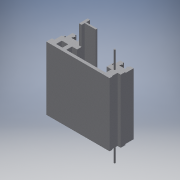
# Autodesk Inventor part: Platform
Saved by Autodesk Inventor 2016 (Build 200138000, 138)
## iProperties
Created: 2015-05-19
Part Number: Platform
Material: Steel
Document SubType Name: Modeling
Designer: Andy
Density: 7.85 g/cm^3
Appearance: Plate
Mass: 10057.4 g
Surface Area: 2204.12 cm^2
Volume: 1281.2 cm^3
Author: Andy
Autodesk Inventor part; units mm, degrees
ref_plane "YZ Plane" through (0, 0, 0) normal (1, 0, 0) x (0, 1, 0)
ref_plane "XZ Plane" through (0, 0, 0) normal (0, 1, 0) x (-1, 0, 0)
sketch "Sketch1" plane through (0, 0, 0) normal (0, 1, 0) x (-1, 0, 0)
  line L0 (0, 0) -> (199, 0)
  line L1 (199, 0) -> (199, 199)
  line L2 (199, 199) -> (0, 199)
  line L3 (0, 199) -> (0, 0)
  dimension "d0" = 199
  dimension "d1" = 199
  constraints: 8 end point, 2 parallel, 1 horizontal, 1 perpendicular
  measures "d0" distance of L0.start L0.end
  measures "d1" distance of L1.end L0.end
extrude "Extrusion1" add sketch "Sketch1" along normal blind 9
sketch "Sketch2" plane through (0, 9, 0) normal (0, 1, 0) x (1, 0, 0)
  line L0 (0, 0) -> (-199, 0) projected
  line L1 (-199, -199) -> (0, -199) projected
  line L2 (0, 0) -> (-2, 0)
  line L3 (-2, 0) -> (-2, -199)
  line L4 (-2, 0) -> (-21, 0)
  line L5 (-21, 0) -> (-21, -199)
  dimension "d4" = 2
  dimension "d5" = 19
  constraints: 8 end point, 4 point on line, 2 perpendicular
  measures "d4" distance of L0.start L2.end
  measures "d5" distance of L2.end L4.end
extrude "Extrusion2" add sketch "Sketch2" along normal blind 18
sketch "Sketch4" plane through (-199, 0, 199) normal (0, 0, 1) x (1, 0, 0)
  line L0 (178, 27) -> (197, 27) projected
  line L1 (197, 27) -> (207, 27)
  line L2 (207, 27) -> (207, 41)
  line L3 (178, 27) -> (163, 27)
  line L4 (163, 27) -> (163, 47)
  line L5 (163, 47) -> (165, 47)
  line L6 (165, 47) -> (165, 41)
  line L7 (165, 41) -> (207, 41)
  dimension "d9" = 10
  dimension "d10" = 14
  dimension "d11" = 15
  dimension "d12" = 20
  dimension "d13" = 2
  constraints: 14 end point, 5 perpendicular, 2 horizontal
  measures "d9" distance of L0.end L1.end
  measures "d10" distance of L1.end L2.end
  measures "d11" distance of L0.start L3.end
  measures "d12" distance of L3.end L4.end
  measures "d13" distance of L4.end L5.end
extrude "Extrusion3" add sketch "Sketch4" against normal blind 199
ref_plane "Work Plane1" through (-199, 0, 196) normal (0, 0, 1) x (1, 0, 0)
sketch "Sketch5" plane through (-199, 0, 196) normal (0, 0, 1) x (1, 0, 0)
  line L0 (165, 41) -> (207, 41)
  line L1 (207, 41) -> (207, 68)
  line L2 (165, 68) -> (165, 41)
  line L3 (176.05, 68) -> (176.05, 64.5)
  line L4 (176.05, 64.5) -> (180.3, 61.2)
  line L5 (195.95, 64.5) -> (191.7, 61.2)
  line L6 (195.95, 64.5) -> (195.95, 68)
  line L7 (195.95, 53) -> (195.95, 54.5)
  line L8 (195.95, 54.5) -> (191.7, 61.2)
  line L9 (176.05, 54.5) -> (180.3, 61.2)
  line L10 (176.05, 53) -> (176.05, 54.5)
  line L11 (195.95, 53) -> (176.05, 53)
  line L12 (207, 68) -> (195.95, 68)
  line L13 (207, 68) -> (195.95, 68)
  line L14 (176.05, 68) -> (165, 68)
  line L15 (15, 41) -> (57, 41)
  line L16 (57, 41) -> (57, 68)
  line L17 (15, 68) -> (15, 41)
  line L18 (26.05, 68) -> (26.05, 64.5)
  line L19 (26.05, 64.5) -> (30.3, 61.2)
  line L20 (45.95, 64.5) -> (41.7, 61.2)
  line L21 (45.95, 64.5) -> (45.95, 68)
  line L22 (45.95, 53) -> (45.95, 54.5)
  line L23 (45.95, 54.5) -> (41.7, 61.2)
  line L24 (26.05, 54.5) -> (30.3, 61.2)
  line L25 (26.05, 53) -> (26.05, 54.5)
  line L26 (45.95, 53) -> (26.05, 53)
  line L27 (57, 68) -> (45.95, 68)
  line L28 (57, 68) -> (45.95, 68)
  line L29 (26.05, 68) -> (15, 68)
  line L30 (0, 9) -> (178, 9) projected
  point P0 (199, 0)
  point P1 (176.05, 51)
  point P2 (26.05, 51)
  dimension "d17" = 27
  dimension "d18" = 1.5
  dimension "d19" = 1.5
  dimension "d20" = 11.05
  dimension "d32" = 27
  dimension "d33" = 1.5
  dimension "d34" = 1.5
  dimension "d35" = 11.05
  dimension "d56" = 32
  constraints: 60 end point, 6 parallel, 3 equal length, 2 horizontal, 2 perpendicular, 1 collinear
  measures "d17" distance of L1.end L0.end
  measures "d18" distance of L7.start L7.end
  measures "d19" distance of L10.start L9.start
  measures "d20" distance of L6.end L1.end
  measures "d32" distance of L27.start L15.end
  measures "d33" distance of L26.start L22.end
  measures "d34" distance of L26.end L25.end
  measures "d35" distance of L27.end L27.start
  measures "d56" distance between parallel lines of L30 L15
extrude "Extrusion4" add sketch "Sketch5" against normal blind 193 contours L2 L14 L3 L4 L9 L10 L11 L7 L8 L5 L6 L12 L1 L0
sketch "Sketch6" plane through (-199, 0, 199) normal (0, 0, 1) x (1, 0, 0)
  line L0 (0, 9) -> (178, 9) projected
  line L1 (0, 9) -> (22, 9)
  line L2 (22, 9) -> (22, 18)
  line L3 (7.723, 18) -> (0, 18)
  line L4 (0, 18) -> (0, 9)
  line L5 (22, 18) -> (22, 27)
  line L6 (22, 41) -> (7.723, 41)
  line L7 (7.723, 41) -> (7.723, 18)
  line L8 (70, 27) -> (70, 41)
  line L9 (70, 41) -> (22, 41)
  line L10 (54, 9) -> (54, 27)
  line L11 (42, 9) -> (42, 27)
  line L12 (22, 27) -> (42, 27)
  line L13 (54, 27) -> (70, 27)
  line L14 (0, 9) -> (22, 9)
  line L15 (42, 9) -> (54, 9)
  dimension "d29" = 20
  dimension "d55" = 14
  dimension "d57" = 18
  constraints: 30 end point, 5 parallel, 5 perpendicular, 2 point on line, 1 collinear
  measures "d29" distance between parallel lines of L2 L11
  measures "d55" distance between parallel lines of L9 L12
  measures "d57" distance between parallel lines of L0 L13
extrude "Extrusion5" add sketch "Sketch6" against normal blind 199 contours L4 L3 L7 L6 L9 L8 L13 L10 L0 L11 L12 L5 L2
sketch "Sketch8" plane through (-199, 0, 196) normal (0, 0, 1) x (1, 0, 0)
  line L0 (207, 41) -> (165, 41) projected
  line L1 (207, 41) -> (207, 68) projected
  line L2 (207, 68) -> (195.95, 68) projected
  line L3 (195.95, 68) -> (195.95, 64.5) projected
  line L4 (195.95, 64.5) -> (191.7, 61.2) projected
  line L5 (191.7, 61.2) -> (195.95, 54.5) projected
  line L6 (195.95, 54.5) -> (195.95, 53) projected
  line L7 (195.95, 53) -> (176.05, 53) projected
  line L8 (176.05, 53) -> (176.05, 54.5) projected
  line L9 (176.05, 54.5) -> (180.3, 61.2) projected
  line L10 (180.3, 61.2) -> (176.05, 64.5) projected
  line L11 (176.05, 64.5) -> (176.05, 68) projected
  line L12 (176.05, 68) -> (165, 68) projected
  line L13 (165, 68) -> (165, 47) projected
  line L14 (165, 41) -> (165, 47) projected
  line L15 (7.723, 41) -> (70, 41) projected
  point P0 (199, 0)
extrude "Extrusion6" add sketch "Sketch5" against normal blind 193 contours L17 L29 L18 L19 L24 L25 L26 L22 L23 L20 L21 L27 L16 L15
sketch "Sketch9" plane through (-199, 0, 199) normal (0, 0, 1) x (1, 0, 0)
  line L0 (70, 41) -> (7.723, 41) projected
  line L1 (57, 41) -> (62, 41)
  line L2 (62, 41) -> (62, 46)
  line L3 (62, 46) -> (57, 46)
  line L4 (57, 46) -> (57, 41)
  line L5 (15, 41) -> (12, 41)
  line L6 (12, 41) -> (12, 46)
  line L7 (12, 46) -> (15, 46)
  line L8 (15, 46) -> (15, 41)
  dimension "d38" = 5
  dimension "d39" = 3
  constraints: 16 end point, 4 parallel, 2 perpendicular, 2 point on line
  measures "d38" distance of L2.end L1.end
  measures "d39" distance of L5.start L5.end
extrude "Extrusion7" add sketch "Sketch9" against normal blind 199
sketch "Sketch10" plane through (-199, 0, 199) normal (0, 0, 1) x (1, 0, 0)
  line L0 (62, 41) -> (62, 46) projected
  line L1 (62, 41) -> (70, 41)
  line L2 (70, 68) -> (62, 68)
  line L3 (62, 68) -> (62, 41)
  line L4 (70, 55.5) -> (105, 55.5)
  line L5 (70, 55.5) -> (105, 55.5)
  line L6 (70, 50.5) -> (105, 50.5)
  line L7 (70, 50.5) -> (105, 50.5)
  line L8 (70, 50.5) -> (105, 50.5)
  line L9 (105, 50.5) -> (105, 55.5)
  line L10 (105, 55.5) -> (70, 55.5)
  line L11 (70, 37) -> (70, 50.5)
  line L12 (70, 55.5) -> (70, 68)
  line L13 (70, 41) -> (70, 50.5)
  line L14 (70, 55.5) -> (70, 68)
  point P0 (0, 0)
  dimension "d42" = 35
  dimension "d59" = 27
  dimension "d60" = 12.5
  dimension "d61" = 5
  constraints: 28 end point, 4 perpendicular, 3 parallel, 1 collinear
  measures "d42" distance of L7.end L7.start
  measures "d59" distance between parallel lines of L2 L1
  measures "d60" distance between parallel lines of L4 L2
  measures "d61" distance between parallel lines of L7 L4
extrude "Extrusion8" add sketch "Sketch10" against normal blind 199
extrude "Extrusion9" add sketch "Sketch10" along normal blind 60
sketch "Sketch11" plane through (-199, 0, 199) normal (0, 0, 1) x (1, 0, 0)
  line L0 (178, 27) -> (183, 27)
  line L1 (183, 27) -> (183, 32)
  circle A0 centre (183, 32) radius 2.5
  dimension "d47" = 5
  dimension "d50" = 5
  constraints: 4 end point, 1 centre point, 1 coincident, 1 horizontal, 1 vertical
  measures "d47" distance of L0.start L0.end
  measures "d50" distance of L0.end L1.end
extrude "Extrusion10" add sketch "Sketch11" along normal blind 55
sketch "Sketch12" plane through (0, 0, 0) normal (0, 0, -1) x (-1, 0, 0)
  circle A0 centre (16, 32) radius 2.5 projected
  circle A1 centre (16, 32) radius 2.5
  constraints: 1 centre point, 1 coincident
extrude "Extrusion11" add sketch "Sketch12" along normal blind 55
body "Solid1"
